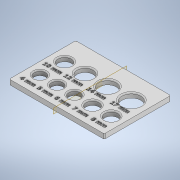
# Autodesk Inventor part: mmHexSocketSetOf9
Saved by Autodesk Inventor 2021 (Build 250183000, 183)
## iProperties
Created: 2020-03-12
Part Number: mmHexSocketSetOf9
Material: Generic
Document SubType Name: Modeling
Designer: robst
Density: 1 g/cm^3
Appearance: Default
Author: robst
Autodesk Inventor part; units mm, degrees
(part 1 of 2)
ref_plane "XZ Plane" through (0, 0, 0) normal (0, 1, 0) x (-1, 0, 0)
ref_plane "XY Plane" through (0, 0, 0) normal (0, 0, 1) x (1, 0, 0)
sketch "Sketch1" plane through (0, 0, 0) normal (0, 1, 0) x (-1, 0, 0)
  line L0 (63.5, 44.45) -> (-63.5, 44.45)
  line L1 (-63.5, 44.45) -> (-63.5, -44.45)
  line L2 (-63.5, -44.45) -> (63.5, -44.45)
  line L3 (63.5, -44.45) -> (63.5, 44.45)
  line L4 (63.5, 44.45) -> (-63.5, -44.45) construction
  line L5 (-63.5, 44.45) -> (63.5, -44.45) construction
  point P0 (0, 0)
  dimension "d3" = 88.9
  dimension "d13" = 127
  constraints: 12 end point, 2 midpoint, 2 parallel, 1 horizontal, 1 perpendicular
  measures "d3" distance of L2.end L0.start
  measures "d13" distance of L1.end L2.end
extrude "Extrusion1" add sketch "Sketch1" against normal blind 6.35
sketch "Sketch4" plane through (0, 0, 0) normal (0, 1, 0) x (1, 0, 0)
  line L0 (-63.5, -44.45) -> (-63.5, 44.45) construction
  line L1 (-63.5, -19.05) -> (63.5, -19.05) construction
  line L2 (63.5, 44.45) -> (63.5, -44.45) construction
  line L3 (-63.5, -44.45) -> (63.5, -44.45) projected
  circle A0 centre (-47.9975, -19.05) radius 7.62
  circle A1 centre (-24.8751, -19.05) radius 7.62
  circle A2 centre (-1.7526, -19.05) radius 7.62
  circle A3 centre (22.3859, -19.05) radius 8.636
  circle A4 centre (47.5403, -19.05) radius 8.636
  line L4 (-63.5, 12.7) -> (63.5, 12.7) construction
  circle A5 centre (-46.736, 12.7) radius 8.89
  circle A6 centre (-19.3675, 12.7) radius 10.6045
  circle A7 centre (10.668, 12.7) radius 11.557
  circle A8 centre (42.6085, 12.7) radius 12.5095
  point P0 (0, 0)
  dimension "d16" = 25.4
  dimension "hex4mmHole" = 15.24
  dimension "gap0" = 7.8825
  dimension "hex5mmHole" = 15.24
  dimension "gap1" = 23.1225
  dimension "hex6mmHole" = 15.24
  dimension "gap2" = 23.1225
  dimension "gap3" = 24.1385
  dimension "gap4" = 25.1545
  dimension "hex7mmHole" = 17.272
  dimension "hex8mmHole" = 17.272
  dimension "d27" = 7.3237
  dimension "frontToBackRowGap" = 31.75
  dimension "gap5" = 7.874
  dimension "hex10mmHole" = 17.78
  dimension "hex12mmHole" = 21.209
  dimension "gap6" = 27.3685
  dimension "hex14mmHole" = 23.114
  dimension "gap7" = 30.0355
  dimension "hex17mmHole" = 25.019
  dimension "gap8" = 31.9405
  dimension "d37" = 8.382
  constraints: 13 point on line, 9 centre point, 4 end point, 1 horizontal, 1 perpendicular
  measures "d16" distance between parallel lines of L1 L3
  measures "hex4mmHole" diameter of A0
  measures "gap0" distance edge to line of A0 L0
  measures "hex5mmHole" diameter of A1
  measures "gap1" distance of A1.centre A0.centre
  measures "hex6mmHole" diameter of A2
  measures "gap2" distance of A2.centre A1.centre
  measures "gap3" distance of A3.centre A2.centre
  measures "gap4" distance of A4.centre A3.centre
  measures "hex7mmHole" diameter of A3
  measures "hex8mmHole" diameter of A4
  measures "d27" distance edge to line of A4 L2
  measures "frontToBackRowGap" distance between parallel lines of L4 L1
  measures "gap5" distance edge to line of A5 L0
  measures "hex10mmHole" diameter of A5
  measures "hex12mmHole" diameter of A6
  measures "gap6" distance of A6.centre A5.centre
  measures "hex14mmHole" diameter of A7
  measures "gap7" distance of A7.centre A6.centre
  measures "hex17mmHole" diameter of A8
  measures "gap8" distance of A8.centre A7.centre
  measures "d37" distance edge to line of A8 L2
extrude "Extrusion3" cut sketch "Sketch4" against normal through all
sketch "Sketch7" plane through (0, 0, 0) normal (0, 1, 0) x (1, 0, 0)
  circle A0 centre (-47.9975, -19.05) radius 7.62 construction
  line L0 (63.5, -44.45) -> (-63.5, -44.45) construction
  line L1 (-55.6175, -35.6779) -> (-40.3775, -35.6779) construction
  line L2 (-32.4951, -35.6779) -> (-17.2551, -35.6779) construction
  line L3 (-9.3726, -35.6779) -> (5.8674, -35.6779) construction
  line L4 (13.7499, -35.6779) -> (30.7679, -35.6779) construction
  line L5 (38.6503, -35.6779) -> (55.6683, -35.6779) construction
  line L6 (-55.626, -3.81) -> (-38.354, -3.81) construction
  line L7 (-30.48, -3.81) -> (-7.62, -3.81) construction
  line L8 (0.254, -3.81) -> (23.114, -3.81) construction
  line L9 (30.988, -3.81) -> (55.626, -3.81) construction
  line L10 (-55.1019, -5.334) -> (-58.4571, -5.334)
  line L11 (-58.4571, -5.334) -> (-58.4571, -4.4489)
  line L12 (-58.4571, -4.4489) -> (-57.3867, -4.4489)
  line L13 (-57.3867, -4.4489) -> (-57.3867, -1.7607)
  line L14 (-57.3867, -1.7607) -> (-58.4571, -1.7607)
  line L15 (-58.4571, -1.7607) -> (-58.4571, -0.9333)
  spline S0 degree 2 poles (-58.4571, -0.9333) (-58.2224, -0.9333) (-57.7572, -0.8715) (-57.6172, -0.8056) knots 0 0 0 1 2 2 2
  spline S1 degree 2 poles (-57.6172, -0.8056) (-57.4567, -0.7233) (-57.2756, -0.4475) (-57.2591, -0.2416) knots 0 0 0 1 2 2 2
  line L16 (-57.2591, -0.2416) -> (-56.1476, -0.2416)
  line L17 (-56.1476, -0.2416) -> (-56.1476, -4.4489)
  line L18 (-56.1476, -4.4489) -> (-55.1019, -4.4489)
  line L19 (-55.1019, -4.4489) -> (-55.1019, -5.334)
  spline S2 degree 2 poles (-50.4912, -2.794) (-50.4912, -3.4527) (-50.7012, -4.4407) (-50.9359, -4.7741) knots 0 0 0 1 2 2 2
  spline S3 degree 2 poles (-50.9359, -4.7741) (-51.1664, -5.1035) (-51.9115, -5.441) (-52.4467, -5.441) knots 0 0 0 1 2 2 2
  spline S4 degree 2 poles (-52.4467, -5.441) (-52.986, -5.441) (-53.727, -5.1035) (-53.9616, -4.7659) knots 0 0 0 1 2 2 2
  spline S5 degree 2 poles (-53.9616, -4.7659) (-54.1963, -4.4324) (-54.4062, -3.4527) (-54.4062, -2.794) knots 0 0 0 1 2 2 2
  spline S6 degree 2 poles (-54.4062, -2.794) (-54.4062, -2.1189) (-54.1963, -1.1638) (-53.9575, -0.818) knots 0 0 0 1 2 2 2
  spline S7 degree 2 poles (-53.9575, -0.818) (-53.7187, -0.4804) (-52.9654, -0.1511) (-52.4467, -0.1511) knots 0 0 0 1 2 2 2
  spline S8 degree 2 poles (-52.4467, -0.1511) (-51.8992, -0.1511) (-51.1664, -0.4969) (-50.9317, -0.8386) knots 0 0 0 1 2 2 2
  spline S9 degree 2 poles (-50.9317, -0.8386) (-50.7012, -1.172) (-50.4912, -2.1559) (-50.4912, -2.794) knots 0 0 0 1 2 2 2
  spline S10 degree 2 poles (-51.7715, -2.794) (-51.7715, -1.8513) (-52.0803, -1.0897) (-52.4467, -1.0897) knots 0 0 0 1 2 2 2
  spline S11 degree 2 poles (-52.4467, -1.0897) (-52.8131, -1.0897) (-53.1259, -1.8513) (-53.1259, -2.7981) knots 0 0 0 1 2 2 2
  spline S12 degree 2 poles (-53.1259, -2.7981) (-53.1259, -3.7285) (-52.8131, -4.5024) (-52.4467, -4.5024) knots 0 0 0 1 2 2 2
  spline S13 degree 2 poles (-52.4467, -4.5024) (-52.0844, -4.5024) (-51.7715, -3.7285) (-51.7715, -2.794) knots 0 0 0 1 2 2 2
  line L20 (-43.1471, -5.334) -> (-43.1471, -3.4197)
  spline S14 degree 2 poles (-43.1471, -3.4197) (-43.1471, -3.1357) (-43.1676, -2.7487) (-43.2171, -2.6252) knots 0 0 0 1 2 2 2
  spline S15 degree 2 poles (-43.2171, -2.6252) (-43.2706, -2.5017) (-43.4846, -2.3906) (-43.6781, -2.3906) knots 0 0 0 1 2 2 2
  spline S16 degree 2 poles (-43.6781, -2.3906) (-43.814, -2.3906) (-44.0774, -2.5099) (-44.2339, -2.6211) knots 0 0 0 1 2 2 2
  line L21 (-44.2339, -2.6211) -> (-44.2339, -5.334)
  line L22 (-44.2339, -5.334) -> (-45.4359, -5.334)
  line L23 (-45.4359, -5.334) -> (-45.4359, -3.4197)
  spline S17 degree 2 poles (-45.4359, -3.4197) (-45.4359, -3.1398) (-45.4606, -2.7487) (-45.51, -2.6252) knots 0 0 0 1 2 2 2
  spline S18 degree 2 poles (-45.51, -2.6252) (-45.5636, -2.5017) (-45.7776, -2.3906) (-45.9711, -2.3906) knots 0 0 0 1 2 2 2
  spline S19 degree 2 poles (-45.9711, -2.3906) (-46.1152, -2.3906) (-46.3993, -2.5264) (-46.531, -2.6211) knots 0 0 0 1 2 2 2
  line L24 (-46.531, -2.6211) -> (-46.531, -5.334)
  line L25 (-46.531, -5.334) -> (-47.7248, -5.334)
  line L26 (-47.7248, -5.334) -> (-47.7248, -1.5014)
  line L27 (-47.7248, -1.5014) -> (-46.531, -1.5014)
  line L28 (-46.531, -1.5014) -> (-46.531, -1.9254)
  spline S20 degree 2 poles (-46.531, -1.9254) (-46.2387, -1.6784) (-45.7159, -1.3984) (-45.3907, -1.3984) knots 0 0 0 1 2 2 2
  spline S21 degree 2 poles (-45.3907, -1.3984) (-45.0407, -1.3984) (-44.5056, -1.7319) (-44.3656, -2.0653) knots 0 0 0 1 2 2 2
  spline S22 degree 2 poles (-44.3656, -2.0653) (-44.0239, -1.7442) (-43.4147, -1.3984) (-43.1018, -1.3984) knots 0 0 0 1 2 2 2
  spline S23 degree 2 poles (-43.1018, -1.3984) (-42.8342, -1.3984) (-42.4102, -1.5672) (-42.2661, -1.7401) knots 0 0 0 1 2 2 2
  spline S24 degree 2 poles (-42.2661, -1.7401) (-42.1055, -1.9254) (-41.945, -2.4317) (-41.945, -2.8393) knots 0 0 0 1 2 2 2
  line L29 (-41.945, -2.8393) -> (-41.945, -5.334)
  line L30 (-41.945, -5.334) -> (-43.1471, -5.334)
  line L31 (-36.4863, -5.334) -> (-36.4863, -3.4197)
  spline S25 degree 2 poles (-36.4863, -3.4197) (-36.4863, -3.1357) (-36.5068, -2.7487) (-36.5562, -2.6252) knots 0 0 0 1 2 2 2
  spline S26 degree 2 poles (-36.5562, -2.6252) (-36.6098, -2.5017) (-36.8238, -2.3906) (-37.0173, -2.3906) knots 0 0 0 1 2 2 2
  spline S27 degree 2 poles (-37.0173, -2.3906) (-37.1532, -2.3906) (-37.4166, -2.5099) (-37.5731, -2.6211) knots 0 0 0 1 2 2 2
  line L32 (-37.5731, -2.6211) -> (-37.5731, -5.334)
  line L33 (-37.5731, -5.334) -> (-38.7751, -5.334)
  line L34 (-38.7751, -5.334) -> (-38.7751, -3.4197)
  spline S28 degree 2 poles (-38.7751, -3.4197) (-38.7751, -3.1398) (-38.7998, -2.7487) (-38.8492, -2.6252) knots 0 0 0 1 2 2 2
  spline S29 degree 2 poles (-38.8492, -2.6252) (-38.9028, -2.5017) (-39.1168, -2.3906) (-39.3103, -2.3906) knots 0 0 0 1 2 2 2
  spline S30 degree 2 poles (-39.3103, -2.3906) (-39.4544, -2.3906) (-39.7384, -2.5264) (-39.8702, -2.6211) knots 0 0 0 1 2 2 2
  line L35 (-39.8702, -2.6211) -> (-39.8702, -5.334)
  line L36 (-39.8702, -5.334) -> (-41.064, -5.334)
  line L37 (-41.064, -5.334) -> (-41.064, -1.5014)
  line L38 (-41.064, -1.5014) -> (-39.8702, -1.5014)
  line L39 (-39.8702, -1.5014) -> (-39.8702, -1.9254)
  spline S31 degree 2 poles (-39.8702, -1.9254) (-39.5779, -1.6784) (-39.0551, -1.3984) (-38.7299, -1.3984) knots 0 0 0 1 2 2 2
  spline S32 degree 2 poles (-38.7299, -1.3984) (-38.3799, -1.3984) (-37.8448, -1.7319) (-37.7048, -2.0653) knots 0 0 0 1 2 2 2
  spline S33 degree 2 poles (-37.7048, -2.0653) (-37.3631, -1.7442) (-36.7538, -1.3984) (-36.441, -1.3984) knots 0 0 0 1 2 2 2
  spline S34 degree 2 poles (-36.441, -1.3984) (-36.1734, -1.3984) (-35.7494, -1.5672) (-35.6053, -1.7401) knots 0 0 0 1 2 2 2
  spline S35 degree 2 poles (-35.6053, -1.7401) (-35.4447, -1.9254) (-35.2842, -2.4317) (-35.2842, -2.8393) knots 0 0 0 1 2 2 2
  line L40 (-35.2842, -2.8393) -> (-35.2842, -5.334)
  line L41 (-35.2842, -5.334) -> (-36.4863, -5.334)
  line L42 (-27.1619, -5.334) -> (-30.5171, -5.334)
  line L43 (-30.5171, -5.334) -> (-30.5171, -4.4489)
  line L44 (-30.5171, -4.4489) -> (-29.4467, -4.4489)
  line L45 (-29.4467, -4.4489) -> (-29.4467, -1.7607)
  line L46 (-29.4467, -1.7607) -> (-30.5171, -1.7607)
  line L47 (-30.5171, -1.7607) -> (-30.5171, -0.9333)
  spline S36 degree 2 poles (-30.5171, -0.9333) (-30.2824, -0.9333) (-29.8172, -0.8715) (-29.6772, -0.8056) knots 0 0 0 1 2 2 2
  spline S37 degree 2 poles (-29.6772, -0.8056) (-29.5167, -0.7233) (-29.3356, -0.4475) (-29.3191, -0.2416) knots 0 0 0 1 2 2 2
  line L48 (-29.3191, -0.2416) -> (-28.2076, -0.2416)
  line L49 (-28.2076, -0.2416) -> (-28.2076, -4.4489)
  line L50 (-28.2076, -4.4489) -> (-27.1619, -4.4489)
  line L51 (-27.1619, -4.4489) -> (-27.1619, -5.334)
  line L52 (-22.4854, -5.334) -> (-26.2192, -5.334)
  line L53 (-26.2192, -5.334) -> (-26.2192, -4.5065)
  spline S38 degree 2 poles (-26.2192, -4.5065) (-25.7458, -4.1278) (-24.9883, -3.4609) (-24.7043, -3.1604) knots 0 0 0 1 2 2 2
  spline S39 degree 2 poles (-24.7043, -3.1604) (-24.3297, -2.7693) (-23.9962, -2.1724) (-23.9962, -1.8595) knots 0 0 0 1 2 2 2
  spline S40 degree 2 poles (-23.9962, -1.8595) (-23.9962, -1.5055) (-24.4202, -1.1267) (-24.799, -1.1267) knots 0 0 0 1 2 2 2
  spline S41 degree 2 poles (-24.799, -1.1267) (-24.9924, -1.1267) (-25.3382, -1.2214) (-25.5153, -1.2955) knots 0 0 0 1 2 2 2
  spline S42 degree 2 poles (-25.5153, -1.2955) (-25.6882, -1.3737) (-25.9352, -1.5384) (-25.9969, -1.5796) knots 0 0 0 1 2 2 2
  line L54 (-25.9969, -1.5796) -> (-26.0957, -1.5796)
  line L55 (-26.0957, -1.5796) -> (-26.0957, -0.4722)
  spline S43 degree 2 poles (-26.0957, -0.4722) (-25.8817, -0.3693) (-24.9677, -0.1552) (-24.5437, -0.1552) knots 0 0 0 1 2 2 2
  spline S44 degree 2 poles (-24.5437, -0.1552) (-23.6381, -0.1552) (-22.7077, -0.9621) (-22.7077, -1.6907) knots 0 0 0 1 2 2 2
  spline S45 degree 2 poles (-22.7077, -1.6907) (-22.7077, -2.1394) (-23.1317, -3.004) (-23.6216, -3.498) knots 0 0 0 1 2 2 2
  spline S46 degree 2 poles (-23.6216, -3.498) (-23.9303, -3.8026) (-24.5108, -4.276) (-24.6384, -4.3748) knots 0 0 0 1 2 2 2
  line L56 (-24.6384, -4.3748) -> (-22.4854, -4.3748)
  line L57 (-22.4854, -4.3748) -> (-22.4854, -5.334)
  line L58 (-15.2071, -5.334) -> (-15.2071, -3.4197)
  spline S47 degree 2 poles (-15.2071, -3.4197) (-15.2071, -3.1357) (-15.2276, -2.7487) (-15.2771, -2.6252) knots 0 0 0 1 2 2 2
  spline S48 degree 2 poles (-15.2771, -2.6252) (-15.3306, -2.5017) (-15.5446, -2.3906) (-15.7381, -2.3906) knots 0 0 0 1 2 2 2
  spline S49 degree 2 poles (-15.7381, -2.3906) (-15.874, -2.3906) (-16.1374, -2.5099) (-16.2939, -2.6211) knots 0 0 0 1 2 2 2
  line L59 (-16.2939, -2.6211) -> (-16.2939, -5.334)
  line L60 (-16.2939, -5.334) -> (-17.4959, -5.334)
  line L61 (-17.4959, -5.334) -> (-17.4959, -3.4197)
  spline S50 degree 2 poles (-17.4959, -3.4197) (-17.4959, -3.1398) (-17.5206, -2.7487) (-17.57, -2.6252) knots 0 0 0 1 2 2 2
  spline S51 degree 2 poles (-17.57, -2.6252) (-17.6236, -2.5017) (-17.8376, -2.3906) (-18.0311, -2.3906) knots 0 0 0 1 2 2 2
  spline S52 degree 2 poles (-18.0311, -2.3906) (-18.1752, -2.3906) (-18.4593, -2.5264) (-18.591, -2.6211) knots 0 0 0 1 2 2 2
  line L62 (-18.591, -2.6211) -> (-18.591, -5.334)
  line L63 (-18.591, -5.334) -> (-19.7848, -5.334)
  line L64 (-19.7848, -5.334) -> (-19.7848, -1.5014)
  line L65 (-19.7848, -1.5014) -> (-18.591, -1.5014)
  line L66 (-18.591, -1.5014) -> (-18.591, -1.9254)
  spline S53 degree 2 poles (-18.591, -1.9254) (-18.2987, -1.6784) (-17.7759, -1.3984) (-17.4507, -1.3984) knots 0 0 0 1 2 2 2
  spline S54 degree 2 poles (-17.4507, -1.3984) (-17.1007, -1.3984) (-16.5656, -1.7319) (-16.4256, -2.0653) knots 0 0 0 1 2 2 2
  spline S55 degree 2 poles (-16.4256, -2.0653) (-16.0839, -1.7442) (-15.4747, -1.3984) (-15.1618, -1.3984) knots 0 0 0 1 2 2 2
  spline S56 degree 2 poles (-15.1618, -1.3984) (-14.8942, -1.3984) (-14.4702, -1.5672) (-14.3261, -1.7401) knots 0 0 0 1 2 2 2
  spline S57 degree 2 poles (-14.3261, -1.7401) (-14.1655, -1.9254) (-14.005, -2.4317) (-14.005, -2.8393) knots 0 0 0 1 2 2 2
  line L67 (-14.005, -2.8393) -> (-14.005, -5.334)
  line L68 (-14.005, -5.334) -> (-15.2071, -5.334)
  line L69 (-8.5463, -5.334) -> (-8.5463, -3.4197)
  spline S58 degree 2 poles (-8.5463, -3.4197) (-8.5463, -3.1357) (-8.5668, -2.7487) (-8.6162, -2.6252) knots 0 0 0 1 2 2 2
  spline S59 degree 2 poles (-8.6162, -2.6252) (-8.6698, -2.5017) (-8.8838, -2.3906) (-9.0773, -2.3906) knots 0 0 0 1 2 2 2
  spline S60 degree 2 poles (-9.0773, -2.3906) (-9.2132, -2.3906) (-9.4766, -2.5099) (-9.6331, -2.6211) knots 0 0 0 1 2 2 2
  line L70 (-9.6331, -2.6211) -> (-9.6331, -5.334)
  line L71 (-9.6331, -5.334) -> (-10.8351, -5.334)
  line L72 (-10.8351, -5.334) -> (-10.8351, -3.4197)
  spline S61 degree 2 poles (-10.8351, -3.4197) (-10.8351, -3.1398) (-10.8598, -2.7487) (-10.9092, -2.6252) knots 0 0 0 1 2 2 2
  spline S62 degree 2 poles (-10.9092, -2.6252) (-10.9628, -2.5017) (-11.1768, -2.3906) (-11.3703, -2.3906) knots 0 0 0 1 2 2 2
  spline S63 degree 2 poles (-11.3703, -2.3906) (-11.5144, -2.3906) (-11.7984, -2.5264) (-11.9302, -2.6211) knots 0 0 0 1 2 2 2
  line L73 (-11.9302, -2.6211) -> (-11.9302, -5.334)
  line L74 (-11.9302, -5.334) -> (-13.124, -5.334)
  line L75 (-13.124, -5.334) -> (-13.124, -1.5014)
  line L76 (-13.124, -1.5014) -> (-11.9302, -1.5014)
  line L77 (-11.9302, -1.5014) -> (-11.9302, -1.9254)
  spline S64 degree 2 poles (-11.9302, -1.9254) (-11.6379, -1.6784) (-11.1151, -1.3984) (-10.7899, -1.3984) knots 0 0 0 1 2 2 2
  spline S65 degree 2 poles (-10.7899, -1.3984) (-10.4399, -1.3984) (-9.9048, -1.7319) (-9.7648, -2.0653) knots 0 0 0 1 2 2 2
  spline S66 degree 2 poles (-9.7648, -2.0653) (-9.4231, -1.7442) (-8.8138, -1.3984) (-8.501, -1.3984) knots 0 0 0 1 2 2 2
  spline S67 degree 2 poles (-8.501, -1.3984) (-8.2334, -1.3984) (-7.8094, -1.5672) (-7.6653, -1.7401) knots 0 0 0 1 2 2 2
  spline S68 degree 2 poles (-7.6653, -1.7401) (-7.5047, -1.9254) (-7.3442, -2.4317) (-7.3442, -2.8393) knots 0 0 0 1 2 2 2
  line L78 (-7.3442, -2.8393) -> (-7.3442, -5.334)
  line L79 (-7.3442, -5.334) -> (-8.5463, -5.334)
  line L80 (3.5721, -5.334) -> (0.2169, -5.334)
  line L81 (0.2169, -5.334) -> (0.2169, -4.4489)
  line L82 (0.2169, -4.4489) -> (1.2873, -4.4489)
  line L83 (1.2873, -4.4489) -> (1.2873, -1.7607)
  line L84 (1.2873, -1.7607) -> (0.2169, -1.7607)
  line L85 (0.2169, -1.7607) -> (0.2169, -0.9333)
  spline S69 degree 2 poles (0.2169, -0.9333) (0.4516, -0.9333) (0.9168, -0.8715) (1.0568, -0.8056) knots 0 0 0 1 2 2 2
  spline S70 degree 2 poles (1.0568, -0.8056) (1.2173, -0.7233) (1.3984, -0.4475) (1.4149, -0.2416) knots 0 0 0 1 2 2 2
  line L86 (1.4149, -0.2416) -> (2.5264, -0.2416)
  line L87 (2.5264, -0.2416) -> (2.5264, -4.4489)
  line L88 (2.5264, -4.4489) -> (3.5721, -4.4489)
  line L89 (3.5721, -4.4489) -> (3.5721, -5.334)
  line L90 (8.3104, -4.1484) -> (7.6229, -4.1484)
  line L91 (7.6229, -4.1484) -> (7.6229, -5.3464)
  line L92 (7.6229, -5.3464) -> (6.392, -5.3464)
  line L93 (6.392, -5.3464) -> (6.392, -4.1484)
  line L94 (6.392, -4.1484) -> (4.1525, -4.1484)
  line L95 (4.1525, -4.1484) -> (4.1525, -3.2016)
  line L96 (4.1525, -3.2016) -> (6.3508, -0.254)
  line L97 (6.3508, -0.254) -> (7.6229, -0.254)
  line L98 (7.6229, -0.254) -> (7.6229, -3.2345)
  line L99 (7.6229, -3.2345) -> (8.3104, -3.2345)
  line L100 (8.3104, -3.2345) -> (8.3104, -4.1484)
  line L101 (6.392, -3.2345) -> (6.392, -1.5055)
  line L102 (6.392, -1.5055) -> (5.1035, -3.2345)
  line L103 (5.1035, -3.2345) -> (6.392, -3.2345)
  line L104 (15.5269, -5.334) -> (15.5269, -3.4197)
  spline S71 degree 2 poles (15.5269, -3.4197) (15.5269, -3.1357) (15.5064, -2.7487) (15.4569, -2.6252) knots 0 0 0 1 2 2 2
  spline S72 degree 2 poles (15.4569, -2.6252) (15.4034, -2.5017) (15.1894, -2.3906) (14.9959, -2.3906) knots 0 0 0 1 2 2 2
  spline S73 degree 2 poles (14.9959, -2.3906) (14.86, -2.3906) (14.5966, -2.5099) (14.4401, -2.6211) knots 0 0 0 1 2 2 2
  line L105 (14.4401, -2.6211) -> (14.4401, -5.334)
  line L106 (14.4401, -5.334) -> (13.2381, -5.334)
  line L107 (13.2381, -5.334) -> (13.2381, -3.4197)
  spline S74 degree 2 poles (13.2381, -3.4197) (13.2381, -3.1398) (13.2134, -2.7487) (13.164, -2.6252) knots 0 0 0 1 2 2 2
  spline S75 degree 2 poles (13.164, -2.6252) (13.1104, -2.5017) (12.8964, -2.3906) (12.7029, -2.3906) knots 0 0 0 1 2 2 2
  spline S76 degree 2 poles (12.7029, -2.3906) (12.5588, -2.3906) (12.2747, -2.5264) (12.143, -2.6211) knots 0 0 0 1 2 2 2
  line L108 (12.143, -2.6211) -> (12.143, -5.334)
  line L109 (12.143, -5.334) -> (10.9492, -5.334)
  line L110 (10.9492, -5.334) -> (10.9492, -1.5014)
  line L111 (10.9492, -1.5014) -> (12.143, -1.5014)
  line L112 (12.143, -1.5014) -> (12.143, -1.9254)
  spline S77 degree 2 poles (12.143, -1.9254) (12.4353, -1.6784) (12.9581, -1.3984) (13.2833, -1.3984) knots 0 0 0 1 2 2 2
  spline S78 degree 2 poles (13.2833, -1.3984) (13.6333, -1.3984) (14.1684, -1.7319) (14.3084, -2.0653) knots 0 0 0 1 2 2 2
  spline S79 degree 2 poles (14.3084, -2.0653) (14.6501, -1.7442) (15.2593, -1.3984) (15.5722, -1.3984) knots 0 0 0 1 2 2 2
  spline S80 degree 2 poles (15.5722, -1.3984) (15.8398, -1.3984) (16.2638, -1.5672) (16.4079, -1.7401) knots 0 0 0 1 2 2 2
  spline S81 degree 2 poles (16.4079, -1.7401) (16.5685, -1.9254) (16.729, -2.4317) (16.729, -2.8393) knots 0 0 0 1 2 2 2
  line L113 (16.729, -2.8393) -> (16.729, -5.334)
  line L114 (16.729, -5.334) -> (15.5269, -5.334)
  line L115 (22.1877, -5.334) -> (22.1877, -3.4197)
  spline S82 degree 2 poles (22.1877, -3.4197) (22.1877, -3.1357) (22.1672, -2.7487) (22.1178, -2.6252) knots 0 0 0 1 2 2 2
  spline S83 degree 2 poles (22.1178, -2.6252) (22.0642, -2.5017) (21.8502, -2.3906) (21.6567, -2.3906) knots 0 0 0 1 2 2 2
  spline S84 degree 2 poles (21.6567, -2.3906) (21.5208, -2.3906) (21.2574, -2.5099) (21.1009, -2.6211) knots 0 0 0 1 2 2 2
  line L116 (21.1009, -2.6211) -> (21.1009, -5.334)
  line L117 (21.1009, -5.334) -> (19.8989, -5.334)
  line L118 (19.8989, -5.334) -> (19.8989, -3.4197)
  spline S85 degree 2 poles (19.8989, -3.4197) (19.8989, -3.1398) (19.8742, -2.7487) (19.8248, -2.6252) knots 0 0 0 1 2 2 2
  spline S86 degree 2 poles (19.8248, -2.6252) (19.7712, -2.5017) (19.5572, -2.3906) (19.3637, -2.3906) knots 0 0 0 1 2 2 2
  spline S87 degree 2 poles (19.3637, -2.3906) (19.2196, -2.3906) (18.9356, -2.5264) (18.8038, -2.6211) knots 0 0 0 1 2 2 2
  line L119 (18.8038, -2.6211) -> (18.8038, -5.334)
  line L120 (18.8038, -5.334) -> (17.61, -5.334)
  line L121 (17.61, -5.334) -> (17.61, -1.5014)
  line L122 (17.61, -1.5014) -> (18.8038, -1.5014)
  line L123 (18.8038, -1.5014) -> (18.8038, -1.9254)
  spline S88 degree 2 poles (18.8038, -1.9254) (19.0961, -1.6784) (19.6189, -1.3984) (19.9441, -1.3984) knots 0 0 0 1 2 2 2
  spline S89 degree 2 poles (19.9441, -1.3984) (20.2941, -1.3984) (20.8292, -1.7319) (20.9692, -2.0653) knots 0 0 0 1 2 2 2
  spline S90 degree 2 poles (20.9692, -2.0653) (21.3109, -1.7442) (21.9202, -1.3984) (22.233, -1.3984) knots 0 0 0 1 2 2 2
  spline S91 degree 2 poles (22.233, -1.3984) (22.5006, -1.3984) (22.9246, -1.5672) (23.0687, -1.7401) knots 0 0 0 1 2 2 2
  spline S92 degree 2 poles (23.0687, -1.7401) (23.2293, -1.9254) (23.3898, -2.4317) (23.3898, -2.8393) knots 0 0 0 1 2 2 2
  line L124 (23.3898, -2.8393) -> (23.3898, -5.334)
  line L125 (23.3898, -5.334) -> (22.1877, -5.334)
  line L126 (35.1951, -5.334) -> (31.8399, -5.334)
  line L127 (31.8399, -5.334) -> (31.8399, -4.4489)
  line L128 (31.8399, -4.4489) -> (32.9103, -4.4489)
  line L129 (32.9103, -4.4489) -> (32.9103, -1.7607)
  line L130 (32.9103, -1.7607) -> (31.8399, -1.7607)
  line L131 (31.8399, -1.7607) -> (31.8399, -0.9333)
  spline S93 degree 2 poles (31.8399, -0.9333) (32.0746, -0.9333) (32.5398, -0.8715) (32.6798, -0.8056) knots 0 0 0 1 2 2 2
  spline S94 degree 2 poles (32.6798, -0.8056) (32.8403, -0.7233) (33.0214, -0.4475) (33.0379, -0.2416) knots 0 0 0 1 2 2 2
  line L132 (33.0379, -0.2416) -> (34.1494, -0.2416)
  line L133 (34.1494, -0.2416) -> (34.1494, -4.4489)
  line L134 (34.1494, -4.4489) -> (35.1951, -4.4489)
  line L135 (35.1951, -4.4489) -> (35.1951, -5.334)
  line L136 (39.7605, -1.2626) -> (37.591, -5.334)
  line L137 (37.591, -5.334) -> (36.1748, -5.334)
  line L138 (36.1748, -5.334) -> (38.4431, -1.2132)
  line L139 (38.4431, -1.2132) -> (36.0225, -1.2132)
  line L140 (36.0225, -1.2132) -> (36.0225, -0.254)
  line L141 (36.0225, -0.254) -> (39.7605, -0.254)
  line L142 (39.7605, -0.254) -> (39.7605, -1.2626)
  line L143 (47.1499, -5.334) -> (47.1499, -3.4197)
  spline S95 degree 2 poles (47.1499, -3.4197) (47.1499, -3.1357) (47.1294, -2.7487) (47.0799, -2.6252) knots 0 0 0 1 2 2 2
  spline S96 degree 2 poles (47.0799, -2.6252) (47.0264, -2.5017) (46.8124, -2.3906) (46.6189, -2.3906) knots 0 0 0 1 2 2 2
  spline S97 degree 2 poles (46.6189, -2.3906) (46.483, -2.3906) (46.2196, -2.5099) (46.0631, -2.6211) knots 0 0 0 1 2 2 2
  line L144 (46.0631, -2.6211) -> (46.0631, -5.334)
  line L145 (46.0631, -5.334) -> (44.8611, -5.334)
  line L146 (44.8611, -5.334) -> (44.8611, -3.4197)
  spline S98 degree 2 poles (44.8611, -3.4197) (44.8611, -3.1398) (44.8364, -2.7487) (44.787, -2.6252) knots 0 0 0 1 2 2 2
  spline S99 degree 2 poles (44.787, -2.6252) (44.7334, -2.5017) (44.5194, -2.3906) (44.3259, -2.3906) knots 0 0 0 1 2 2 2
  spline S100 degree 2 poles (44.3259, -2.3906) (44.1818, -2.3906) (43.8977, -2.5264) (43.766, -2.6211) knots 0 0 0 1 2 2 2
  line L147 (43.766, -2.6211) -> (43.766, -5.334)
  line L148 (43.766, -5.334) -> (42.5722, -5.334)
  line L149 (42.5722, -5.334) -> (42.5722, -1.5014)
  line L150 (42.5722, -1.5014) -> (43.766, -1.5014)
  line L151 (43.766, -1.5014) -> (43.766, -1.9254)
  spline S101 degree 2 poles (43.766, -1.9254) (44.0583, -1.6784) (44.5811, -1.3984) (44.9063, -1.3984) knots 0 0 0 1 2 2 2
  spline S102 degree 2 poles (44.9063, -1.3984) (45.2563, -1.3984) (45.7914, -1.7319) (45.9314, -2.0653) knots 0 0 0 1 2 2 2
  spline S103 degree 2 poles (45.9314, -2.0653) (46.2731, -1.7442) (46.8823, -1.3984) (47.1952, -1.3984) knots 0 0 0 1 2 2 2
  spline S104 degree 2 poles (47.1952, -1.3984) (47.4628, -1.3984) (47.8868, -1.5672) (48.0309, -1.7401) knots 0 0 0 1 2 2 2
  spline S105 degree 2 poles (48.0309, -1.7401) (48.1915, -1.9254) (48.352, -2.4317) (48.352, -2.8393) knots 0 0 0 1 2 2 2
  line L152 (48.352, -2.8393) -> (48.352, -5.334)
  line L153 (48.352, -5.334) -> (47.1499, -5.334)
  line L154 (53.8107, -5.334) -> (53.8107, -3.4197)
  spline S106 degree 2 poles (53.8107, -3.4197) (53.8107, -3.1357) (53.7902, -2.7487) (53.7408, -2.6252) knots 0 0 0 1 2 2 2
  spline S107 degree 2 poles (53.7408, -2.6252) (53.6872, -2.5017) (53.4732, -2.3906) (53.2797, -2.3906) knots 0 0 0 1 2 2 2
  spline S108 degree 2 poles (53.2797, -2.3906) (53.1438, -2.3906) (52.8804, -2.5099) (52.7239, -2.6211) knots 0 0 0 1 2 2 2
  line L155 (52.7239, -2.6211) -> (52.7239, -5.334)
  line L156 (52.7239, -5.334) -> (51.5219, -5.334)
  line L157 (51.5219, -5.334) -> (51.5219, -3.4197)
  spline S109 degree 2 poles (51.5219, -3.4197) (51.5219, -3.1398) (51.4972, -2.7487) (51.4478, -2.6252) knots 0 0 0 1 2 2 2
  spline S110 degree 2 poles (51.4478, -2.6252) (51.3942, -2.5017) (51.1802, -2.3906) (50.9867, -2.3906) knots 0 0 0 1 2 2 2
  spline S111 degree 2 poles (50.9867, -2.3906) (50.8426, -2.3906) (50.5586, -2.5264) (50.4268, -2.6211) knots 0 0 0 1 2 2 2
  line L158 (50.4268, -2.6211) -> (50.4268, -5.334)
  line L159 (50.4268, -5.334) -> (49.233, -5.334)
  line L160 (49.233, -5.334) -> (49.233, -1.5014)
  line L161 (49.233, -1.5014) -> (50.4268, -1.5014)
  line L162 (50.4268, -1.5014) -> (50.4268, -1.9254)
  spline S112 degree 2 poles (50.4268, -1.9254) (50.7191, -1.6784) (51.2419, -1.3984) (51.5671, -1.3984) knots 0 0 0 1 2 2 2
  spline S113 degree 2 poles (51.5671, -1.3984) (51.9171, -1.3984) (52.4522, -1.7319) (52.5922, -2.0653) knots 0 0 0 1 2 2 2
  spline S114 degree 2 poles (52.5922, -2.0653) (52.9339, -1.7442) (53.5432, -1.3984) (53.856, -1.3984) knots 0 0 0 1 2 2 2
  spline S115 degree 2 poles (53.856, -1.3984) (54.1236, -1.3984) (54.5476, -1.5672) (54.6917, -1.7401) knots 0 0 0 1 2 2 2
  spline S116 degree 2 poles (54.6917, -1.7401) (54.8523, -1.9254) (55.0128, -2.4317) (55.0128, -2.8393) knots 0 0 0 1 2 2 2
  line L163 (55.0128, -2.8393) -> (55.0128, -5.334)
  line L164 (55.0128, -5.334) -> (53.8107, -5.334)
  line L165 (-53.5962, -36.0163) -> (-54.2837, -36.0163)
  line L166 (-54.2837, -36.0163) -> (-54.2837, -37.2142)
  line L167 (-54.2837, -37.2142) -> (-55.5146, -37.2142)
  line L168 (-55.5146, -37.2142) -> (-55.5146, -36.0163)
  line L169 (-55.5146, -36.0163) -> (-57.7541, -36.0163)
  line L170 (-57.7541, -36.0163) -> (-57.7541, -35.0694)
  line L171 (-57.7541, -35.0694) -> (-55.5558, -32.1219)
  line L172 (-55.5558, -32.1219) -> (-54.2837, -32.1219)
  line L173 (-54.2837, -32.1219) -> (-54.2837, -35.1024)
  line L174 (-54.2837, -35.1024) -> (-53.5962, -35.1024)
  line L175 (-53.5962, -35.1024) -> (-53.5962, -36.0163)
  line L176 (-55.5146, -35.1024) -> (-55.5146, -33.3733)
  line L177 (-55.5146, -33.3733) -> (-56.8031, -35.1024)
  line L178 (-56.8031, -35.1024) -> (-55.5146, -35.1024)
  line L179 (-46.3797, -37.2019) -> (-46.3797, -35.2876)
  spline S117 degree 2 poles (-46.3797, -35.2876) (-46.3797, -35.0036) (-46.4003, -34.6166) (-46.4497, -34.4931) knots 0 0 0 1 2 2 2
  spline S118 degree 2 poles (-46.4497, -34.4931) (-46.5032, -34.3696) (-46.7172, -34.2584) (-46.9107, -34.2584) knots 0 0 0 1 2 2 2
  spline S119 degree 2 poles (-46.9107, -34.2584) (-47.0466, -34.2584) (-47.31, -34.3778) (-47.4665, -34.489) knots 0 0 0 1 2 2 2
  line L180 (-47.4665, -34.489) -> (-47.4665, -37.2019)
  line L181 (-47.4665, -37.2019) -> (-48.6686, -37.2019)
  line L182 (-48.6686, -37.2019) -> (-48.6686, -35.2876)
  spline S120 degree 2 poles (-48.6686, -35.2876) (-48.6686, -35.0077) (-48.6933, -34.6166) (-48.7427, -34.4931) knots 0 0 0 1 2 2 2
  spline S121 degree 2 poles (-48.7427, -34.4931) (-48.7962, -34.3696) (-49.0102, -34.2584) (-49.2037, -34.2584) knots 0 0 0 1 2 2 2
  spline S122 degree 2 poles (-49.2037, -34.2584) (-49.3478, -34.2584) (-49.6319, -34.3943) (-49.7636, -34.489) knots 0 0 0 1 2 2 2
  line L183 (-49.7636, -34.489) -> (-49.7636, -37.2019)
  line L184 (-49.7636, -37.2019) -> (-50.9574, -37.2019)
  line L185 (-50.9574, -37.2019) -> (-50.9574, -33.3692)
  line L186 (-50.9574, -33.3692) -> (-49.7636, -33.3692)
  line L187 (-49.7636, -33.3692) -> (-49.7636, -33.7932)
  spline S123 degree 2 poles (-49.7636, -33.7932) (-49.4713, -33.5462) (-48.9485, -33.2663) (-48.6233, -33.2663) knots 0 0 0 1 2 2 2
  spline S124 degree 2 poles (-48.6233, -33.2663) (-48.2734, -33.2663) (-47.7382, -33.5998) (-47.5982, -33.9332) knots 0 0 0 1 2 2 2
  spline S125 degree 2 poles (-47.5982, -33.9332) (-47.2565, -33.6121) (-46.6473, -33.2663) (-46.3344, -33.2663) knots 0 0 0 1 2 2 2
  spline S126 degree 2 poles (-46.3344, -33.2663) (-46.0668, -33.2663) (-45.6428, -33.4351) (-45.4987, -33.608) knots 0 0 0 1 2 2 2
  spline S127 degree 2 poles (-45.4987, -33.608) (-45.3381, -33.7932) (-45.1776, -34.2996) (-45.1776, -34.7072) knots 0 0 0 1 2 2 2
  line L188 (-45.1776, -34.7072) -> (-45.1776, -37.2019)
  line L189 (-45.1776, -37.2019) -> (-46.3797, -37.2019)
  line L190 (-39.7189, -37.2019) -> (-39.7189, -35.2876)
  spline S128 degree 2 poles (-39.7189, -35.2876) (-39.7189, -35.0036) (-39.7394, -34.6166) (-39.7888, -34.4931) knots 0 0 0 1 2 2 2
  spline S129 degree 2 poles (-39.7888, -34.4931) (-39.8424, -34.3696) (-40.0564, -34.2584) (-40.2499, -34.2584) knots 0 0 0 1 2 2 2
  spline S130 degree 2 poles (-40.2499, -34.2584) (-40.3858, -34.2584) (-40.6492, -34.3778) (-40.8057, -34.489) knots 0 0 0 1 2 2 2
  line L191 (-40.8057, -34.489) -> (-40.8057, -37.2019)
  line L192 (-40.8057, -37.2019) -> (-42.0077, -37.2019)
  line L193 (-42.0077, -37.2019) -> (-42.0077, -35.2876)
  spline S131 degree 2 poles (-42.0077, -35.2876) (-42.0077, -35.0077) (-42.0324, -34.6166) (-42.0818, -34.4931) knots 0 0 0 1 2 2 2
  spline S132 degree 2 poles (-42.0818, -34.4931) (-42.1354, -34.3696) (-42.3494, -34.2584) (-42.5429, -34.2584) knots 0 0 0 1 2 2 2
  spline S133 degree 2 poles (-42.5429, -34.2584) (-42.687, -34.2584) (-42.971, -34.3943) (-43.1028, -34.489) knots 0 0 0 1 2 2 2
  line L194 (-43.1028, -34.489) -> (-43.1028, -37.2019)
  line L195 (-43.1028, -37.2019) -> (-44.2966, -37.2019)
  line L196 (-44.2966, -37.2019) -> (-44.2966, -33.3692)
  line L197 (-44.2966, -33.3692) -> (-43.1028, -33.3692)
  line L198 (-43.1028, -33.3692) -> (-43.1028, -33.7932)
  spline S134 degree 2 poles (-43.1028, -33.7932) (-42.8105, -33.5462) (-42.2877, -33.2663) (-41.9625, -33.2663) knots 0 0 0 1 2 2 2
  spline S135 degree 2 poles (-41.9625, -33.2663) (-41.6125, -33.2663) (-41.0774, -33.5998) (-40.9374, -33.9332) knots 0 0 0 1 2 2 2
  spline S136 degree 2 poles (-40.9374, -33.9332) (-40.5957, -33.6121) (-39.9864, -33.2663) (-39.6736, -33.2663) knots 0 0 0 1 2 2 2
  spline S137 degree 2 poles (-39.6736, -33.2663) (-39.406, -33.2663) (-38.982, -33.4351) (-38.8379, -33.608) knots 0 0 0 1 2 2 2
  spline S138 degree 2 poles (-38.8379, -33.608) (-38.6773, -33.7932) (-38.5168, -34.2996) (-38.5168, -34.7072) knots 0 0 0 1 2 2 2
  line L199 (-38.5168, -34.7072) -> (-38.5168, -37.2019)
  line L200 (-38.5168, -37.2019) -> (-39.7189, -37.2019)
  spline S139 degree 2 poles (-30.6508, -35.4811) (-30.6508, -35.8804) (-30.9225, -36.5555) (-31.1901, -36.7984) knots 0 0 0 1 2 2 2
  spline S140 degree 2 poles (-31.1901, -36.7984) (-31.4577, -37.0413) (-32.1904, -37.3089) (-32.7256, -37.3089) knots 0 0 0 1 2 2 2
  spline S141 degree 2 poles (-32.7256, -37.3089) (-33.2937, -37.3048) (-34.1088, -37.1195) (-34.3764, -37.0001) knots 0 0 0 1 2 2 2
  line L201 (-34.3764, -37.0001) -> (-34.3764, -35.8928)
  line L202 (-34.3764, -35.8928) -> (-34.2611, -35.8928)
  spline S142 degree 2 poles (-34.2611, -35.8928) (-34.1623, -35.9463) (-33.9236, -36.0862) (-33.7301, -36.1603) knots 0 0 0 1 2 2 2
  spline S143 degree 2 poles (-33.7301, -36.1603) (-33.5489, -36.2303) (-33.1743, -36.325) (-32.9479, -36.325) knots 0 0 0 1 2 2 2
  spline S144 degree 2 poles (-32.9479, -36.325) (-32.7503, -36.325) (-32.2892, -36.2262) (-32.1493, -36.0945) knots 0 0 0 1 2 2 2
  spline S145 degree 2 poles (-32.1493, -36.0945) (-32.0463, -35.9916) (-31.9311, -35.7404) (-31.9311, -35.5305) knots 0 0 0 1 2 2 2
  spline S146 degree 2 poles (-31.9311, -35.5305) (-31.9311, -35.3494) (-32.0793, -35.0941) (-32.1987, -35.0159) knots 0 0 0 1 2 2 2
  spline S147 degree 2 poles (-32.1987, -35.0159) (-32.3716, -34.9006) (-32.8656, -34.8348) (-33.0426, -34.8348) knots 0 0 0 1 2 2 2
  spline S148 degree 2 poles (-33.0426, -34.8348) (-33.3225, -34.8348) (-33.8536, -34.9253) (-34.0471, -34.9747) knots 0 0 0 1 2 2 2
  line L203 (-34.0471, -34.9747) -> (-34.1582, -34.9747)
  line L204 (-34.1582, -34.9747) -> (-34.1582, -32.1219)
  line L205 (-34.1582, -32.1219) -> (-30.7908, -32.1219)
  line L206 (-30.7908, -32.1219) -> (-30.7908, -33.0811)
  line L207 (-30.7908, -33.0811) -> (-32.952, -33.0811)
  line L208 (-32.952, -33.0811) -> (-32.952, -33.925)
  spline S149 degree 2 poles (-32.952, -33.925) (-32.8491, -33.9167) (-32.5651, -33.9085) (-32.4868, -33.9085) knots 0 0 0 1 2 2 2
  spline S150 degree 2 poles (-32.4868, -33.9085) (-32.1204, -33.9085) (-31.5029, -34.0567) (-31.2601, -34.209) knots 0 0 0 1 2 2 2
  spline S151 degree 2 poles (-31.2601, -34.209) (-30.9719, -34.3984) (-30.6508, -35.0283) (-30.6508, -35.4811) knots 0 0 0 1 2 2 2
  line L209 (-23.2572, -37.2019) -> (-23.2572, -35.2876)
  spline S152 degree 2 poles (-23.2572, -35.2876) (-23.2572, -35.0036) (-23.2778, -34.6166) (-23.3272, -34.4931) knots 0 0 0 1 2 2 2
  spline S153 degree 2 poles (-23.3272, -34.4931) (-23.3807, -34.3696) (-23.5948, -34.2584) (-23.7883, -34.2584) knots 0 0 0 1 2 2 2
  spline S154 degree 2 poles (-23.7883, -34.2584) (-23.9241, -34.2584) (-24.1876, -34.3778) (-24.344, -34.489) knots 0 0 0 1 2 2 2
  line L210 (-24.344, -34.489) -> (-24.344, -37.2019)
  line L211 (-24.344, -37.2019) -> (-25.5461, -37.2019)
  line L212 (-25.5461, -37.2019) -> (-25.5461, -35.2876)
  spline S155 degree 2 poles (-25.5461, -35.2876) (-25.5461, -35.0077) (-25.5708, -34.6166) (-25.6202, -34.4931) knots 0 0 0 1 2 2 2
  spline S156 degree 2 poles (-25.6202, -34.4931) (-25.6737, -34.3696) (-25.8878, -34.2584) (-26.0813, -34.2584) knots 0 0 0 1 2 2 2
  spline S157 degree 2 poles (-26.0813, -34.2584) (-26.2253, -34.2584) (-26.5094, -34.3943) (-26.6411, -34.489) knots 0 0 0 1 2 2 2
  line L213 (-26.6411, -34.489) -> (-26.6411, -37.2019)
  line L214 (-26.6411, -37.2019) -> (-27.835, -37.2019)
  line L215 (-27.835, -37.2019) -> (-27.835, -33.3692)
  line L216 (-27.835, -33.3692) -> (-26.6411, -33.3692)
  line L217 (-26.6411, -33.3692) -> (-26.6411, -33.7932)
  spline S158 degree 2 poles (-26.6411, -33.7932) (-26.3488, -33.5462) (-25.826, -33.2663) (-25.5008, -33.2663) knots 0 0 0 1 2 2 2
  spline S159 degree 2 poles (-25.5008, -33.2663) (-25.1509, -33.2663) (-24.6157, -33.5998) (-24.4757, -33.9332) knots 0 0 0 1 2 2 2
  spline S160 degree 2 poles (-24.4757, -33.9332) (-24.1341, -33.6121) (-23.5248, -33.2663) (-23.2119, -33.2663) knots 0 0 0 1 2 2 2
  spline S161 degree 2 poles (-23.2119, -33.2663) (-22.9443, -33.2663) (-22.5203, -33.4351) (-22.3762, -33.608) knots 0 0 0 1 2 2 2
  spline S162 degree 2 poles (-22.3762, -33.608) (-22.2157, -33.7932) (-22.0551, -34.2996) (-22.0551, -34.7072) knots 0 0 0 1 2 2 2
  line L218 (-22.0551, -34.7072) -> (-22.0551, -37.2019)
  line L219 (-22.0551, -37.2019) -> (-23.2572, -37.2019)
  line L220 (-16.5964, -37.2019) -> (-16.5964, -35.2876)
  spline S163 degree 2 poles (-16.5964, -35.2876) (-16.5964, -35.0036) (-16.617, -34.6166) (-16.6664, -34.4931) knots 0 0 0 1 2 2 2
  spline S164 degree 2 poles (-16.6664, -34.4931) (-16.7199, -34.3696) (-16.934, -34.2584) (-17.1274, -34.2584) knots 0 0 0 1 2 2 2
  spline S165 degree 2 poles (-17.1274, -34.2584) (-17.2633, -34.2584) (-17.5268, -34.3778) (-17.6832, -34.489) knots 0 0 0 1 2 2 2
  line L221 (-17.6832, -34.489) -> (-17.6832, -37.2019)
  line L222 (-17.6832, -37.2019) -> (-18.8853, -37.2019)
  line L223 (-18.8853, -37.2019) -> (-18.8853, -35.2876)
  spline S166 degree 2 poles (-18.8853, -35.2876) (-18.8853, -35.0077) (-18.91, -34.6166) (-18.9594, -34.4931) knots 0 0 0 1 2 2 2
  spline S167 degree 2 poles (-18.9594, -34.4931) (-19.0129, -34.3696) (-19.227, -34.2584) (-19.4204, -34.2584) knots 0 0 0 1 2 2 2
  spline S168 degree 2 poles (-19.4204, -34.2584) (-19.5645, -34.2584) (-19.8486, -34.3943) (-19.9803, -34.489) knots 0 0 0 1 2 2 2
  line L224 (-19.9803, -34.489) -> (-19.9803, -37.2019)
  line L225 (-19.9803, -37.2019) -> (-21.1742, -37.2019)
  line L226 (-21.1742, -37.2019) -> (-21.1742, -33.3692)
  line L227 (-21.1742, -33.3692) -> (-19.9803, -33.3692)
  line L228 (-19.9803, -33.3692) -> (-19.9803, -33.7932)
  spline S169 degree 2 poles (-19.9803, -33.7932) (-19.688, -33.5462) (-19.1652, -33.2663) (-18.84, -33.2663) knots 0 0 0 1 2 2 2
  spline S170 degree 2 poles (-18.84, -33.2663) (-18.4901, -33.2663) (-17.9549, -33.5998) (-17.8149, -33.9332) knots 0 0 0 1 2 2 2
  spline S171 degree 2 poles (-17.8149, -33.9332) (-17.4733, -33.6121) (-16.864, -33.2663) (-16.5511, -33.2663) knots 0 0 0 1 2 2 2
  spline S172 degree 2 poles (-16.5511, -33.2663) (-16.2835, -33.2663) (-15.8595, -33.4351) (-15.7154, -33.608) knots 0 0 0 1 2 2 2
  spline S173 degree 2 poles (-15.7154, -33.608) (-15.5549, -33.7932) (-15.3943, -34.2996) (-15.3943, -34.7072) knots 0 0 0 1 2 2 2
  line L229 (-15.3943, -34.7072) -> (-15.3943, -37.2019)
  line L230 (-15.3943, -37.2019) -> (-16.5964, -37.2019)
  spline S174 degree 2 poles (-7.4419, -35.4729) (-7.4419, -36.2756) (-8.4587, -37.3089) (-9.3479, -37.3089) knots 0 0 0 1 2 2 2
  spline S175 degree 2 poles (-9.3479, -37.3089) (-9.7925, -37.3089) (-10.4882, -37.0537) (-10.7311, -36.8025) knots 0 0 0 1 2 2 2
  spline S176 degree 2 poles (-10.7311, -36.8025) (-11.0193, -36.5103) (-11.328, -35.584) (-11.328, -34.9377) knots 0 0 0 1 2 2 2
  spline S177 degree 2 poles (-11.328, -34.9377) (-11.328, -34.2708) (-11.0399, -33.2334) (-10.7146, -32.8341) knots 0 0 0 1 2 2 2
  spline S178 degree 2 poles (-10.7146, -32.8341) (-10.4059, -32.4553) (-9.4014, -32.0272) (-8.7139, -32.0272) knots 0 0 0 1 2 2 2
  spline S179 degree 2 poles (-8.7139, -32.0272) (-8.4628, -32.0272) (-7.9606, -32.0931) (-7.87, -32.1136) knots 0 0 0 1 2 2 2
  line L231 (-7.87, -32.1136) -> (-7.87, -33.1099)
  line L232 (-7.87, -33.1099) -> (-7.9606, -33.1099)
  spline S180 degree 2 poles (-7.9606, -33.1099) (-8.0511, -33.0646) (-8.4628, -32.9534) (-8.7263, -32.9534) knots 0 0 0 1 2 2 2
  spline S181 degree 2 poles (-8.7263, -32.9534) (-9.3232, -32.9534) (-9.9736, -33.5833) (-10.0519, -34.1679) knots 0 0 0 1 2 2 2
  spline S182 degree 2 poles (-10.0519, -34.1679) (-9.8007, -34.0073) (-9.2861, -33.8179) (-8.9609, -33.8179) knots 0 0 0 1 2 2 2
  spline S183 degree 2 poles (-8.9609, -33.8179) (-8.6851, -33.8179) (-8.2035, -33.9661) (-8.0182, -34.1061) knots 0 0 0 1 2 2 2
  spline S184 degree 2 poles (-8.0182, -34.1061) (-7.7547, -34.3078) (-7.4419, -34.9624) (-7.4419, -35.4729) knots 0 0 0 1 2 2 2
  spline S185 degree 2 poles (-8.928, -36.2386) (-8.8292, -36.1151) (-8.7222, -35.8269) (-8.7222, -35.5346) knots 0 0 0 1 2 2 2
  spline S186 degree 2 poles (-8.7222, -35.5346) (-8.7222, -35.2876) (-8.8457, -34.9665) (-8.9568, -34.8718) knots 0 0 0 1 2 2 2
  spline S187 degree 2 poles (-8.9568, -34.8718) (-9.0721, -34.773) (-9.3561, -34.703) (-9.5167, -34.703) knots 0 0 0 1 2 2 2
  spline S188 degree 2 poles (-9.5167, -34.703) (-9.6525, -34.703) (-9.9325, -34.773) (-10.056, -34.8224) knots 0 0 0 1 2 2 2
  spline S189 degree 2 poles (-10.056, -34.8224) (-10.056, -34.8554) (-10.0642, -35.0118) (-10.0642, -35.1312) knots 0 0 0 1 2 2 2
  spline S190 degree 2 poles (-10.0642, -35.1312) (-10.0642, -35.5717) (-9.9119, -36.1027) (-9.7925, -36.2386) knots 0 0 0 1 2 2 2
  spline S191 degree 2 poles (-9.7925, -36.2386) (-9.7061, -36.3497) (-9.4755, -36.4444) (-9.352, -36.4444) knots 0 0 0 1 2 2 2
  spline S192 degree 2 poles (-9.352, -36.4444) (-9.2491, -36.4444) (-9.0103, -36.3415) (-8.928, -36.2386) knots 0 0 0 1 2 2 2
  line L233 (-0.1347, -37.2019) -> (-0.1347, -35.2876)
  spline S193 degree 2 poles (-0.1347, -35.2876) (-0.1347, -35.0036) (-0.1553, -34.6166) (-0.2047, -34.4931) knots 0 0 0 1 2 2 2
  spline S194 degree 2 poles (-0.2047, -34.4931) (-0.2582, -34.3696) (-0.4723, -34.2584) (-0.6658, -34.2584) knots 0 0 0 1 2 2 2
  spline S195 degree 2 poles (-0.6658, -34.2584) (-0.8016, -34.2584) (-1.0651, -34.3778) (-1.2215, -34.489) knots 0 0 0 1 2 2 2
  line L234 (-1.2215, -34.489) -> (-1.2215, -37.2019)
  line L235 (-1.2215, -37.2019) -> (-2.4236, -37.2019)
  line L236 (-2.4236, -37.2019) -> (-2.4236, -35.2876)
  spline S196 degree 2 poles (-2.4236, -35.2876) (-2.4236, -35.0077) (-2.4483, -34.6166) (-2.4977, -34.4931) knots 0 0 0 1 2 2 2
  spline S197 degree 2 poles (-2.4977, -34.4931) (-2.5512, -34.3696) (-2.7653, -34.2584) (-2.9588, -34.2584) knots 0 0 0 1 2 2 2
  spline S198 degree 2 poles (-2.9588, -34.2584) (-3.1029, -34.2584) (-3.3869, -34.3943) (-3.5187, -34.489) knots 0 0 0 1 2 2 2
  line L237 (-3.5187, -34.489) -> (-3.5187, -37.2019)
  line L238 (-3.5187, -37.2019) -> (-4.7125, -37.2019)
  line L239 (-4.7125, -37.2019) -> (-4.7125, -33.3692)
  line L240 (-4.7125, -33.3692) -> (-3.5187, -33.3692)
  line L241 (-3.5187, -33.3692) -> (-3.5187, -33.7932)
  spline S199 degree 2 poles (-3.5187, -33.7932) (-3.2264, -33.5462) (-2.7036, -33.2663) (-2.3783, -33.2663) knots 0 0 0 1 2 2 2
  spline S200 degree 2 poles (-2.3783, -33.2663) (-2.0284, -33.2663) (-1.4932, -33.5998) (-1.3533, -33.9332) knots 0 0 0 1 2 2 2
  spline S201 degree 2 poles (-1.3533, -33.9332) (-1.0116, -33.6121) (-0.4023, -33.2663) (-0.0895, -33.2663) knots 0 0 0 1 2 2 2
  spline S202 degree 2 poles (-0.0895, -33.2663) (0.1781, -33.2663) (0.6021, -33.4351) (0.7462, -33.608) knots 0 0 0 1 2 2 2
  spline S203 degree 2 poles (0.7462, -33.608) (0.9068, -33.7932) (1.0673, -34.2996) (1.0673, -34.7072) knots 0 0 0 1 2 2 2
  line L242 (1.0673, -34.7072) -> (1.0673, -37.2019)
  line L243 (1.0673, -37.2019) -> (-0.1347, -37.2019)
  line L244 (6.5261, -37.2019) -> (6.5261, -35.2876)
  spline S204 degree 2 poles (6.5261, -35.2876) (6.5261, -35.0036) (6.5055, -34.6166) (6.4561, -34.4931) knots 0 0 0 1 2 2 2
  spline S205 degree 2 poles (6.4561, -34.4931) (6.4026, -34.3696) (6.1885, -34.2584) (5.995, -34.2584) knots 0 0 0 1 2 2 2
  spline S206 degree 2 poles (5.995, -34.2584) (5.8592, -34.2584) (5.5957, -34.3778) (5.4393, -34.489) knots 0 0 0 1 2 2 2
  line L245 (5.4393, -34.489) -> (5.4393, -37.2019)
  line L246 (5.4393, -37.2019) -> (4.2372, -37.2019)
  line L247 (4.2372, -37.2019) -> (4.2372, -35.2876)
  spline S207 degree 2 poles (4.2372, -35.2876) (4.2372, -35.0077) (4.2125, -34.6166) (4.1631, -34.4931) knots 0 0 0 1 2 2 2
  spline S208 degree 2 poles (4.1631, -34.4931) (4.1096, -34.3696) (3.8955, -34.2584) (3.702, -34.2584) knots 0 0 0 1 2 2 2
  spline S209 degree 2 poles (3.702, -34.2584) (3.5579, -34.2584) (3.2739, -34.3943) (3.1421, -34.489) knots 0 0 0 1 2 2 2
  line L248 (3.1421, -34.489) -> (3.1421, -37.2019)
  line L249 (3.1421, -37.2019) -> (1.9483, -37.2019)
  line L250 (1.9483, -37.2019) -> (1.9483, -33.3692)
  line L251 (1.9483, -33.3692) -> (3.1421, -33.3692)
  line L252 (3.1421, -33.3692) -> (3.1421, -33.7932)
  spline S210 degree 2 poles (3.1421, -33.7932) (3.4344, -33.5462) (3.9573, -33.2663) (4.2825, -33.2663) knots 0 0 0 1 2 2 2
  spline S211 degree 2 poles (4.2825, -33.2663) (4.6324, -33.2663) (5.1676, -33.5998) (5.3075, -33.9332) knots 0 0 0 1 2 2 2
  spline S212 degree 2 poles (5.3075, -33.9332) (5.6492, -33.6121) (6.2585, -33.2663) (6.5714, -33.2663) knots 0 0 0 1 2 2 2
  spline S213 degree 2 poles (6.5714, -33.2663) (6.8389, -33.2663) (7.263, -33.4351) (7.407, -33.608) knots 0 0 0 1 2 2 2
  spline S214 degree 2 poles (7.407, -33.608) (7.5676, -33.7932) (7.7281, -34.2996) (7.7281, -34.7072) knots 0 0 0 1 2 2 2
  line L253 (7.7281, -34.7072) -> (7.7281, -37.2019)
  line L254 (7.7281, -37.2019) -> (6.5261, -37.2019)
  line L255 (16.4873, -33.1305) -> (14.3178, -37.2019)
  line L256 (14.3178, -37.2019) -> (12.9016, -37.2019)
  line L257 (12.9016, -37.2019) -> (15.1699, -33.0811)
  line L258 (15.1699, -33.0811) -> (12.7493, -33.0811)
  line L259 (12.7493, -33.0811) -> (12.7493, -32.1219)
  line L260 (12.7493, -32.1219) -> (16.4873, -32.1219)
  line L261 (16.4873, -32.1219) -> (16.4873, -33.1305)
  line L262 (23.8767, -37.2019) -> (23.8767, -35.2876)
  spline S215 degree 2 poles (23.8767, -35.2876) (23.8767, -35.0036) (23.8561, -34.6166) (23.8067, -34.4931) knots 0 0 0 1 2 2 2
  spline S216 degree 2 poles (23.8067, -34.4931) (23.7532, -34.3696) (23.5392, -34.2584) (23.3457, -34.2584) knots 0 0 0 1 2 2 2
  spline S217 degree 2 poles (23.3457, -34.2584) (23.2098, -34.2584) (22.9464, -34.3778) (22.7899, -34.489) knots 0 0 0 1 2 2 2
  line L263 (22.7899, -34.489) -> (22.7899, -37.2019)
  line L264 (22.7899, -37.2019) -> (21.5878, -37.2019)
  line L265 (21.5878, -37.2019) -> (21.5878, -35.2876)
  spline S218 degree 2 poles (21.5878, -35.2876) (21.5878, -35.0077) (21.5631, -34.6166) (21.5137, -34.4931) knots 0 0 0 1 2 2 2
  spline S219 degree 2 poles (21.5137, -34.4931) (21.4602, -34.3696) (21.2462, -34.2584) (21.0527, -34.2584) knots 0 0 0 1 2 2 2
  spline S220 degree 2 poles (21.0527, -34.2584) (20.9086, -34.2584) (20.6245, -34.3943) (20.4928, -34.489) knots 0 0 0 1 2 2 2
  line L266 (20.4928, -34.489) -> (20.4928, -37.2019)
  line L267 (20.4928, -37.2019) -> (19.299, -37.2019)
  line L268 (19.299, -37.2019) -> (19.299, -33.3692)
  line L269 (19.299, -33.3692) -> (20.4928, -33.3692)
  line L270 (20.4928, -33.3692) -> (20.4928, -33.7932)
  spline S221 degree 2 poles (20.4928, -33.7932) (20.7851, -33.5462) (21.3079, -33.2663) (21.6331, -33.2663) knots 0 0 0 1 2 2 2
  spline S222 degree 2 poles (21.6331, -33.2663) (21.983, -33.2663) (22.5182, -33.5998) (22.6582, -33.9332) knots 0 0 0 1 2 2 2
  spline S223 degree 2 poles (22.6582, -33.9332) (22.9999, -33.6121) (23.6091, -33.2663) (23.922, -33.2663) knots 0 0 0 1 2 2 2
  spline S224 degree 2 poles (23.922, -33.2663) (24.1896, -33.2663) (24.6136, -33.4351) (24.7577, -33.608) knots 0 0 0 1 2 2 2
  spline S225 degree 2 poles (24.7577, -33.608) (24.9183, -33.7932) (25.0788, -34.2996) (25.0788, -34.7072) knots 0 0 0 1 2 2 2
  line L271 (25.0788, -34.7072) -> (25.0788, -37.2019)
  line L272 (25.0788, -37.2019) -> (23.8767, -37.2019)
  line L273 (30.5375, -37.2019) -> (30.5375, -35.2876)
  spline S226 degree 2 poles (30.5375, -35.2876) (30.5375, -35.0036) (30.517, -34.6166) (30.4676, -34.4931) knots 0 0 0 1 2 2 2
  spline S227 degree 2 poles (30.4676, -34.4931) (30.414, -34.3696) (30.2, -34.2584) (30.0065, -34.2584) knots 0 0 0 1 2 2 2
  spline S228 degree 2 poles (30.0065, -34.2584) (29.8706, -34.2584) (29.6072, -34.3778) (29.4507, -34.489) knots 0 0 0 1 2 2 2
  line L274 (29.4507, -34.489) -> (29.4507, -37.2019)
  line L275 (29.4507, -37.2019) -> (28.2487, -37.2019)
  line L276 (28.2487, -37.2019) -> (28.2487, -35.2876)
  spline S229 degree 2 poles (28.2487, -35.2876) (28.2487, -35.0077) (28.224, -34.6166) (28.1746, -34.4931) knots 0 0 0 1 2 2 2
  spline S230 degree 2 poles (28.1746, -34.4931) (28.121, -34.3696) (27.907, -34.2584) (27.7135, -34.2584) knots 0 0 0 1 2 2 2
  spline S231 degree 2 poles (27.7135, -34.2584) (27.5694, -34.2584) (27.2854, -34.3943) (27.1536, -34.489) knots 0 0 0 1 2 2 2
  line L277 (27.1536, -34.489) -> (27.1536, -37.2019)
  line L278 (27.1536, -37.2019) -> (25.9598, -37.2019)
  line L279 (25.9598, -37.2019) -> (25.9598, -33.3692)
  line L280 (25.9598, -33.3692) -> (27.1536, -33.3692)
  line L281 (27.1536, -33.3692) -> (27.1536, -33.7932)
  spline S232 degree 2 poles (27.1536, -33.7932) (27.4459, -33.5462) (27.9687, -33.2663) (28.2939, -33.2663) knots 0 0 0 1 2 2 2
  spline S233 degree 2 poles (28.2939, -33.2663) (28.6439, -33.2663) (29.179, -33.5998) (29.319, -33.9332) knots 0 0 0 1 2 2 2
  spline S234 degree 2 poles (29.319, -33.9332) (29.6607, -33.6121) (30.27, -33.2663) (30.5828, -33.2663) knots 0 0 0 1 2 2 2
  spline S235 degree 2 poles (30.5828, -33.2663) (30.8504, -33.2663) (31.2744, -33.4351) (31.4185, -33.608) knots 0 0 0 1 2 2 2
  spline S236 degree 2 poles (31.4185, -33.608) (31.5791, -33.7932) (31.7396, -34.2996) (31.7396, -34.7072) knots 0 0 0 1 2 2 2
  line L282 (31.7396, -34.7072) -> (31.7396, -37.2019)
  line L283 (31.7396, -37.2019) -> (30.5375, -37.2019)
  spline S237 degree 2 poles (41.4865, -35.7898) (41.4865, -36.1151) (41.2148, -36.679) (40.9555, -36.8849) knots 0 0 0 1 2 2 2
  spline S238 degree 2 poles (40.9555, -36.8849) (40.6961, -37.0907) (39.951, -37.3213) (39.4693, -37.3213) knots 0 0 0 1 2 2 2
  spline S239 degree 2 poles (39.4693, -37.3213) (38.9548, -37.3213) (38.1849, -37.0866) (37.9379, -36.8849) knots 0 0 0 1 2 2 2